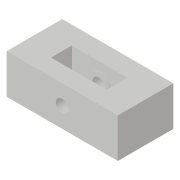
# Autodesk Inventor part: pulley enclosure test
Saved by Autodesk Inventor 2018 (Build 220112000, 112)
## iProperties
Created: 2019-10-04
Part Number: pulley enclosure test
Material: Generic
Document SubType Name: Modeling
Designer: ball
Density: 1 g/cm^3
Appearance: Default
Author: ball
Autodesk Inventor part; units mm, degrees
ref_plane "YZ Plane" through (0, 0, 0) normal (1, 0, 0) x (0, 1, 0)
ref_plane "XZ Plane" through (0, 0, 0) normal (0, 1, 0) x (-1, 0, 0)
ref_plane "XY Plane" through (0, 0, 0) normal (0, 0, 1) x (1, 0, 0)
sketch "Sketch1" plane through (0, 0, 0) normal (0, 1, 0) x (-1, 0, 0)
  line L0 (0, 0) -> (25.4, 0)
  line L1 (25.4, 0) -> (25.4, -12.7)
  line L2 (25.4, -12.7) -> (0, -12.7)
  line L3 (0, -12.7) -> (0, 0)
  line L4 (6.35, -3.81) -> (19.05, -3.81)
  line L5 (19.05, -3.81) -> (19.05, -8.5598)
  line L6 (19.05, -8.5598) -> (6.35, -8.5598)
  line L7 (6.35, -8.5598) -> (6.35, -3.81)
  dimension "d0" = 25.4
  dimension "d1" = 12.7
  dimension "d2" = 12.7
  dimension "d3" = 4.7498
  dimension "d5" = 6.35
  dimension "d6" = 3.81
  constraints: 16 end point, 4 parallel, 2 horizontal, 2 perpendicular
  measures "d0" distance of L1.end L2.end
  measures "d1" distance of L0.end L1.end
  measures "d2" distance of L5.end L6.end
  measures "d3" distance of L4.end L5.end
  measures "d5" distance between parallel lines of L3 L7
  measures "d6" distance between parallel lines of L0 L4
extrude "Extrusion1" add sketch "Sketch1" along normal blind 9
sketch "Sketch2" plane through (-19.05, 0, -8.5598) normal (0, 0, 1) x (1, 0, 0)
  circle A0 centre (6.35, 4.5) radius 2.54
  line L0 (12.7, 0) -> (12.7, 9) projected
  point P0 (19.05, 0)
  dimension "d9" = 5.08
  dimension "d10" = 4.5
  dimension "d11" = 6.35
  constraints: 1 centre point
  measures "d9" diameter of A0
  measures "d10" vertical distance of L0.end A0.centre
  measures "d11" distance from line of L0 A0.centre
extrude "Extrusion2" add sketch "Sketch2" along normal blind 0.1905
sketch "Sketch3" plane through (-6.35, 0, -3.81) normal (0, 0, -1) x (-1, 0, 0)
  circle A0 centre (6.35, 4.5) radius 2.54
  line L0 (0, 0) -> (0, 9) projected
  point P0 (-6.35, 0)
  dimension "d14" = 5.08
  dimension "d15" = 4.5
  dimension "d16" = 6.35
  constraints: 1 centre point
  measures "d14" diameter of A0
  measures "d15" vertical distance of L0.start A0.centre
  measures "d16" distance from line of L0 A0.centre
extrude "Extrusion3" add sketch "Sketch3" along normal blind 0.1905
sketch "Sketch4" plane through (0, 0, -12.7) normal (0, 0, -1) x (-1, 0, 0)
  circle A0 centre (12.7, 4.5) radius 1.4605
  line L0 (0, 0) -> (0, 9) projected
  line L1 (25.4, 0) -> (0, 0) projected
  dimension "d19" = 2.921
  dimension "d20" = 12.7
  dimension "d21" = 4.5
  constraints: 1 centre point
  measures "d19" diameter of A0
  measures "d20" distance from line of L0 A0.centre
  measures "d21" distance from line of L1 A0.centre
hole "Hole1" at (-12.7, 4.5, -12.7) direction (0, 0, 1) diameter 2.921 end through all
body "Solid1"
